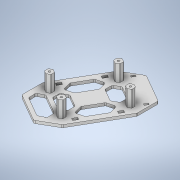
# Autodesk Inventor part: top_body
Saved by Autodesk Inventor 2022 (Build 260153000, 153)
## iProperties
Created: 2022-01-21
Part Number: top_body
Material: Generic
Document SubType Name: Modeling
Designer: felix
Density: 1 g/cm^3
Appearance: Default
Author: felix
Autodesk Inventor part; units mm, degrees
ref_plane "YZ Plane" through (0, 0, 0) normal (1, 0, 0) x (0, 1, 0)
ref_plane "XZ Plane" through (0, 0, 0) normal (0, 1, 0) x (-1, 0, 0)
ref_plane "XY Plane" through (0, 0, 0) normal (0, 0, 1) x (1, 0, 0)
sketch "Sketch1" plane through (0, 0, 0) normal (0, 1, 0) x (-1, 0, 0)
  line L0 (-6.75, 41.2984) -> (6.75, 41.2984)
  line L1 (-8.75, 41.2984) -> (-12.4382, 41.2984)
  line L2 (10.8532, 42.2984) -> (27.4545, 71.0527)
  line L3 (39.1431, 45.1348) -> (-87.6719, 118.3514) construction
  line L4 (27.4545, 73.0527) -> (16.6748, 91.7237)
  line L5 (-8.2836, 49.4226) -> (11.7164, 84.0636) construction
  line L6 (11.7164, 84.0636) -> (-40.2452, 114.0636) construction
  line L7 (-40.2452, 114.0636) -> (-60.2452, 79.4226) construction
  line L8 (-60.2452, 79.4226) -> (-8.2836, 49.4226) construction
  line L9 (27.4545, 73.0527) -> (16.6748, 91.7237)
  line L10 (-13.4382, 41.5663) -> (-38.9549, 56.2984)
  line L11 (15.9428, 92.4557) -> (-9.5739, 107.1878)
  line L12 (-38.9549, 56.2984) -> (-9.5739, 107.1878) construction
  line L13 (8.75, 41.2984) -> (9.1212, 41.2984)
  line L14 (6.75, 41.2984) -> (8.75, 41.2984)
  line L15 (-6.75, 41.2984) -> (-8.75, 41.2984)
  line L16 (-68.0477, 76.6887) -> (-74.7977, 88.38)
  line L17 (-67.0477, 74.9566) -> (-65.2036, 71.7625)
  line L18 (-75.9833, 92.4335) -> (-59.3918, 121.1708)
  line L19 (-57.6613, 122.1708) -> (-36.0921, 122.1878)
  line L20 (-57.6613, 122.1708) -> (-36.0921, 122.1878)
  line L21 (-64.4716, 71.0304) -> (-38.9549, 56.2984)
  line L22 (-35.0906, 121.9198) -> (-9.5739, 107.1878)
  line L23 (-75.7977, 90.1121) -> (-75.9833, 90.4335)
  line L24 (-74.7977, 88.38) -> (-75.7977, 90.1121)
  line L25 (-68.0477, 76.6887) -> (-67.0477, 74.9566)
  line L26 (-41.8469, 122.123) -> (-39.8469, 122.123)
  line L27 (8.363, 47.7877) -> (2.3891, 47.4404)
  line L28 (0.4859, 48.5393) -> (-2.2004, 53.8865)
  line L29 (-2.1453, 55.7843) -> (9.2761, 75.5668)
  line L30 (10.8921, 76.5634) -> (16.8661, 76.9107)
  line L31 (18.7693, 75.8118) -> (21.4556, 70.4646)
  line L32 (21.4005, 68.5668) -> (9.979, 48.7843)
  line L33 (-53.5554, 79.7095) -> (-54.9988, 77.2095)
  line L34 (-55.8648, 76.7095) -> (-58.7516, 76.7095)
  line L35 (-59.6176, 77.2095) -> (-61.061, 79.7095)
  line L36 (-61.061, 80.7095) -> (-59.6176, 83.2095)
  line L37 (-58.7516, 83.7095) -> (-55.8648, 83.7095)
  line L38 (-54.9988, 83.2095) -> (-53.5554, 80.7095)
  circle A0 centre (-57.3082, 80.2095) radius 1.15
  line L39 (-37.1488, 108.1266) -> (-35.7054, 110.6266)
  line L40 (-35.7054, 111.6266) -> (-37.1488, 114.1266)
  line L41 (-38.0148, 114.6266) -> (-40.9016, 114.6266)
  line L42 (-41.7676, 114.1266) -> (-43.211, 111.6266)
  line L43 (-43.211, 110.6266) -> (-41.7676, 108.1266)
  line L44 (-40.9016, 107.6266) -> (-38.0148, 107.6266)
  circle A1 centre (-39.4582, 111.1266) radius 1.15
  line L45 (-11.38, 55.3595) -> (-12.8234, 52.8595)
  line L46 (-12.8234, 51.8595) -> (-11.38, 49.3595)
  line L47 (-10.514, 48.8595) -> (-7.6272, 48.8595)
  line L48 (-6.7612, 49.3595) -> (-5.3178, 51.8595)
  line L49 (-5.3178, 52.8595) -> (-6.7612, 55.3595)
  line L50 (-7.6272, 55.8595) -> (-10.514, 55.8595)
  circle A2 centre (-9.0706, 52.3595) radius 1.15
  line L51 (11.0888, 86.2766) -> (12.5322, 83.7766)
  line L52 (7.336, 86.7766) -> (10.2228, 86.7766)
  line L53 (5.0266, 83.7766) -> (6.47, 86.2766)
  circle A3 centre (8.7794, 83.2766) radius 1.15
  line L54 (12.5322, 82.7766) -> (11.0888, 80.2766)
  line L55 (10.2228, 79.7766) -> (7.336, 79.7766)
  line L56 (6.47, 80.2766) -> (5.0266, 82.7766)
  line L57 (-55.4509, 69.7264) -> (-53.9509, 72.3245)
  line L58 (-53.9509, 72.3245) -> (-49.6208, 69.8245)
  line L59 (-49.6208, 69.8245) -> (-51.1208, 67.2264)
  line L60 (-51.1208, 67.2264) -> (-55.4509, 69.7264)
  line L61 (-29.4509, 114.7598) -> (-30.9509, 112.1617)
  line L62 (-30.9509, 112.1617) -> (-26.6208, 109.6617)
  line L63 (-26.6208, 109.6617) -> (-25.1208, 112.2598)
  line L64 (-25.1208, 112.2598) -> (-29.4509, 114.7598)
  line L65 (-19.0779, 48.7264) -> (-17.5779, 51.3245)
  line L66 (-17.5779, 51.3245) -> (-21.908, 53.8245)
  line L67 (-21.908, 53.8245) -> (-23.408, 51.2264)
  line L68 (-23.408, 51.2264) -> (-19.0779, 48.7264)
  line L69 (2.592, 96.2598) -> (6.9221, 93.7598)
  line L70 (1.092, 93.6617) -> (2.592, 96.2598)
  line L71 (5.4221, 91.1617) -> (1.092, 93.6617)
  line L72 (6.9221, 93.7598) -> (5.4221, 91.1617)
  line L73 (-46.6597, 74.1249) -> (-44.8296, 67.2947)
  line L74 (-43.8977, 66.0803) -> (-28.0121, 56.9088)
  line L75 (-26.4945, 56.709) -> (-19.6643, 58.5391)
  line L76 (-18.2501, 60.9886) -> (-20.0802, 67.8187)
  line L77 (-21.0121, 69.0331) -> (-36.8977, 78.2047)
  line L78 (-38.4154, 78.4045) -> (-45.2455, 76.5744)
  line L79 (18.179, 76.987) -> (1.0762, 47.3641) construction
  line L80 (-47.6152, 61.2984) -> (-30.8618, 90.3161) construction
  line L81 (-30.2946, 51.2984) -> (-13.5413, 80.3161) construction
  line L82 (12.9012, 45.8456) -> (-2.6846, 54.8502) construction
  line L83 (12.8818, 45.8145) -> (-2.6017, 54.7601) construction
  line L84 (-28.8645, 104.9471) -> (-22.0343, 106.7772)
  line L85 (-20.5167, 106.5774) -> (-4.6311, 97.4059)
  line L86 (-3.6992, 96.1914) -> (-1.8691, 89.3613)
  line L87 (-3.2833, 86.9118) -> (-10.1134, 85.0817)
  line L88 (-11.6311, 85.2815) -> (-27.5167, 94.4531)
  line L89 (-28.4486, 95.6675) -> (-30.2787, 102.4976)
  line L90 (-18.2341, 112.1878) -> (-34.9875, 83.1701) construction
  line L91 (-0.9136, 102.1878) -> (-17.667, 73.1701) construction
  line L92 (-57.3082, 80.2095) -> (8.7794, 83.2766) construction
  line L93 (-9.0706, 52.3595) -> (-39.4582, 111.1266) construction
  line L94 (-17.7325, 59.0567) -> (-47.1773, 76.0567) construction
  line L95 (-1.3515, 87.4295) -> (-30.7963, 104.4295) construction
  line L96 (-52.6301, 88.8824) -> (-40.5057, 81.8824) construction
  line L97 (-44.6301, 102.7388) -> (-32.5057, 95.7388) construction
  line L98 (-36.5978, 102.6513) -> (-48.5381, 81.97) construction
  line L99 (3.5167, 73.5911) -> (-3.3141, 61.76)
  line L100 (-5.0679, 60.7601) -> (-10.8053, 60.8227)
  line L101 (-12.5045, 61.8037) -> (-15.4274, 66.7411)
  line L102 (-15.4384, 68.76) -> (-8.6077, 80.5911)
  line L103 (-6.8538, 81.591) -> (-1.1165, 81.5284)
  line L104 (0.5828, 80.5474) -> (3.5057, 75.6099)
  line L105 (-3.8987, 60.7473) -> (-16.0231, 67.7473) construction
  line L106 (4.1013, 74.6038) -> (-8.0231, 81.6038) construction
  line L107 (0.0093, 81.5162) -> (-11.931, 60.8349) construction
  arc A4 (-57.6613, 122.1708) -> (-59.3918, 121.1708) centre (-57.6598, 120.1708) ccw
  arc A5 (-75.9833, 92.4335) -> (-75.9833, 90.4335) centre (-74.2513, 91.4335) ccw
  arc A6 (-35.0906, 121.9198) -> (-36.0921, 122.1878) centre (-36.0906, 120.1878) ccw
  arc A7 (16.6748, 91.7237) -> (15.9428, 92.4557) centre (14.9428, 90.7237) ccw
  arc A8 (27.4545, 71.0527) -> (27.4545, 73.0527) centre (25.7225, 72.0527) ccw
  arc A9 (9.1212, 41.2984) -> (10.8532, 42.2984) centre (9.1212, 43.2984) ccw
  arc A10 (-13.4382, 41.5663) -> (-12.4382, 41.2984) centre (-12.4382, 43.2984) ccw
  arc A11 (-65.2036, 71.7625) -> (-64.4716, 71.0304) centre (-63.4716, 72.7625) ccw
  arc A12 (-61.061, 80.7095) -> (-61.061, 79.7095) centre (-60.195, 80.2095) ccw
  arc A13 (-58.7516, 83.7095) -> (-59.6176, 83.2095) centre (-58.7516, 82.7095) ccw
  arc A14 (-54.9988, 83.2095) -> (-55.8648, 83.7095) centre (-55.8648, 82.7095) ccw
  arc A15 (-53.5554, 79.7095) -> (-53.5554, 80.7095) centre (-54.4215, 80.2095) ccw
  arc A16 (-55.8648, 76.7095) -> (-54.9988, 77.2095) centre (-55.8648, 77.7095) ccw
  arc A17 (-59.6176, 77.2095) -> (-58.7516, 76.7095) centre (-58.7516, 77.7095) ccw
  arc A18 (-43.211, 111.6266) -> (-43.211, 110.6266) centre (-42.345, 111.1266) ccw
  arc A19 (-40.9016, 114.6266) -> (-41.7676, 114.1266) centre (-40.9016, 113.6266) ccw
  arc A20 (-37.1488, 114.1266) -> (-38.0148, 114.6266) centre (-38.0148, 113.6266) ccw
  arc A21 (-35.7054, 110.6266) -> (-35.7054, 111.6266) centre (-36.5715, 111.1266) ccw
  arc A22 (-38.0148, 107.6266) -> (-37.1488, 108.1266) centre (-38.0148, 108.6266) ccw
  arc A23 (-41.7676, 108.1266) -> (-40.9016, 107.6266) centre (-40.9016, 108.6266) ccw
  arc A24 (7.336, 86.7766) -> (6.47, 86.2766) centre (7.336, 85.7766) ccw
  arc A25 (11.0888, 86.2766) -> (10.2228, 86.7766) centre (10.2228, 85.7766) ccw
  arc A26 (12.5322, 82.7766) -> (12.5322, 83.7766) centre (11.6662, 83.2766) ccw
  arc A27 (10.2228, 79.7766) -> (11.0888, 80.2766) centre (10.2228, 80.7766) ccw
  arc A28 (6.47, 80.2766) -> (7.336, 79.7766) centre (7.336, 80.7766) ccw
  arc A29 (5.0266, 83.7766) -> (5.0266, 82.7766) centre (5.8927, 83.2766) ccw
  arc A30 (-12.8234, 52.8595) -> (-12.8234, 51.8595) centre (-11.9573, 52.3595) ccw
  arc A31 (-11.38, 49.3595) -> (-10.514, 48.8595) centre (-10.514, 49.8595) ccw
  arc A32 (-7.6272, 48.8595) -> (-6.7612, 49.3595) centre (-7.6272, 49.8595) ccw
  arc A33 (-5.3178, 51.8595) -> (-5.3178, 52.8595) centre (-6.1838, 52.3595) ccw
  arc A34 (-6.7612, 55.3595) -> (-7.6272, 55.8595) centre (-7.6272, 54.8595) ccw
  arc A35 (-10.514, 55.8595) -> (-11.38, 55.3595) centre (-10.514, 54.8595) ccw
  arc A36 (-45.2455, 76.5744) -> (-46.6597, 74.1249) centre (-44.7278, 74.6425) ccw
  arc A37 (-36.8977, 78.2047) -> (-38.4154, 78.4045) centre (-37.8977, 76.4726) ccw
  arc A38 (-44.8296, 67.2947) -> (-43.8977, 66.0803) centre (-42.8977, 67.8124) ccw
  arc A39 (-28.0121, 56.9088) -> (-26.4945, 56.709) centre (-27.0121, 58.6408) ccw
  arc A40 (-19.6643, 58.5391) -> (-18.2501, 60.9886) centre (-20.182, 60.4709) ccw
  arc A41 (-20.0802, 67.8187) -> (-21.0121, 69.0331) centre (-22.0121, 67.3011) ccw
  arc A42 (-28.4486, 95.6675) -> (-27.5167, 94.4531) centre (-26.5167, 96.1851) ccw
  arc A43 (-28.8645, 104.9471) -> (-30.2787, 102.4976) centre (-28.3468, 103.0153) ccw
  arc A44 (-20.5167, 106.5774) -> (-22.0343, 106.7772) centre (-21.5167, 104.8454) ccw
  arc A45 (-3.6992, 96.1914) -> (-4.6311, 97.4059) centre (-5.6311, 95.6738) ccw
  arc A46 (-3.2833, 86.9118) -> (-1.8691, 89.3613) centre (-3.801, 88.8437) ccw
  arc A47 (-11.6311, 85.2815) -> (-10.1134, 85.0817) centre (-10.6311, 87.0136) ccw
  arc A48 (-2.1453, 55.7843) -> (-2.2004, 53.8865) centre (-0.4133, 54.7843) ccw
  arc A49 (10.8921, 76.5634) -> (9.2761, 75.5668) centre (11.0082, 74.5668) ccw
  arc A50 (18.7693, 75.8118) -> (16.8661, 76.9107) centre (16.9821, 74.914) ccw
  arc A51 (21.4005, 68.5668) -> (21.4556, 70.4646) centre (19.6684, 69.5668) ccw
  arc A52 (8.363, 47.7877) -> (9.979, 48.7843) centre (8.247, 49.7843) ccw
  arc A53 (0.4859, 48.5393) -> (2.3891, 47.4404) centre (2.273, 49.4371) ccw
  arc A54 (-15.4384, 68.76) -> (-15.4274, 66.7411) centre (-13.7064, 67.76) ccw
  arc A55 (-6.8538, 81.591) -> (-8.6077, 80.5911) centre (-6.8756, 79.5911) ccw
  arc A56 (0.5828, 80.5474) -> (-1.1165, 81.5284) centre (-1.1383, 79.5286) ccw
  arc A57 (3.5167, 73.5911) -> (3.5057, 75.6099) centre (1.7846, 74.5911) ccw
  arc A58 (-5.0679, 60.7601) -> (-3.3141, 61.76) centre (-5.0461, 62.76) ccw
  arc A59 (-12.5045, 61.8037) -> (-10.8053, 60.8227) centre (-10.7835, 62.8225) ccw
  line L108 (-45.2147, 101.7262) -> (-52.0455, 89.8951)
  line L109 (-52.0345, 87.8762) -> (-49.1116, 82.9388)
  line L110 (-47.4123, 81.9577) -> (-41.675, 81.8952)
  line L111 (-37.7235, 102.6635) -> (-43.4609, 102.7261)
  line L112 (-33.1014, 96.745) -> (-36.0243, 101.6825)
  line L113 (-39.9211, 82.8951) -> (-33.0904, 94.7262)
  arc A60 (-41.675, 81.8952) -> (-39.9211, 82.8951) centre (-41.6532, 83.8951) ccw
  arc A61 (-33.0904, 94.7262) -> (-33.1014, 96.745) centre (-34.8224, 95.7262) ccw
  arc A62 (-36.0243, 101.6825) -> (-37.7235, 102.6635) centre (-37.7453, 100.6636) ccw
  arc A63 (-43.4609, 102.7261) -> (-45.2147, 101.7262) centre (-43.4827, 100.7262) ccw
  arc A64 (-52.0455, 89.8951) -> (-52.0345, 87.8762) centre (-50.3134, 88.8951) ccw
  arc A65 (-49.1116, 82.9388) -> (-47.4123, 81.9577) centre (-47.3905, 83.9576) ccw
  point P0 (10.2759, 41.2984)
  point P1 (-12.9741, 41.2984)
  point P2 (28.0319, 72.0527)
  point P3 (19.1539, 56.6755)
  point P4 (-67.6827, 106.8106)
  point P5 (-8.2836, 49.4226)
  point P6 (-24.2644, 81.7431)
  point P7 (9.4398, 47.8502)
  point P8 (21.9398, 69.5009)
  point P9 (-53.2668, 80.2095)
  point P10 (-55.2875, 76.7095)
  point P11 (-59.3289, 76.7095)
  point P12 (-61.3497, 80.2095)
  point P13 (-59.3289, 83.7095)
  point P14 (-55.2875, 83.7095)
  point P15 (-37.4375, 107.6266)
  point P16 (-35.4168, 111.1266)
  point P17 (-37.4375, 114.6266)
  point P18 (-41.4789, 114.6266)
  point P19 (-43.4997, 111.1266)
  point P20 (-41.4789, 107.6266)
  point P21 (-11.0913, 55.8595)
  point P22 (-13.112, 52.3595)
  point P23 (-11.0913, 48.8595)
  point P24 (-7.0499, 48.8595)
  point P25 (-5.0291, 52.3595)
  point P26 (-7.0499, 55.8595)
  point P27 (10.8001, 86.7766)
  point P28 (12.8209, 83.2766)
  point P29 (6.7587, 86.7766)
  point P30 (4.738, 83.2766)
  point P31 (10.8001, 79.7766)
  point P32 (6.7587, 79.7766)
  point P33 (-44.6152, 66.4945)
  point P34 (-27.2946, 56.4945)
  point P35 (-20.2946, 68.6189)
  point P36 (-37.6152, 78.6189)
  point P37 (-21.2341, 106.9916)
  point P38 (-3.9136, 96.9916)
  point P39 (-10.9136, 84.8673)
  point P40 (-28.2341, 94.8673)
  dimension "d82" = 23.25
  dimension "d88" = 120
  dimension "d89" = 120
  dimension "d90" = 35.512
  dimension "d91" = 17.756
  dimension "d92" = 17.756
  dimension "d95" = 40
  dimension "d97" = 20
  dimension "d99" = 30
  dimension "d102" = 60
  dimension "d145" = 180
  dimension "d146" = 30
  dimension "d147" = 8.1242
  dimension "d148" = 8.1242
  dimension "d155" = 2.3
  dimension "d156" = 7
  dimension "d160" = 3
  dimension "d162" = 3
  dimension "d163" = 9
  dimension "d169" = 6
  dimension "d170" = 10
  dimension "d171" = 20
  dimension "d172" = 14
  dimension "d179" = 7
  dimension "d181" = 2
  dimension "d186" = 1
  dimension "d187" = 1
  dimension "d189" = 2
  dimension "d190" = 2
  dimension "d191" = 4
  dimension "d192" = 16
  dimension "d193" = 8
  dimension "d194" = 14
  dimension "d195" = 8
  dimension "d204" = 14
  dimension "d206" = 18.762
  dimension "d207" = 28.2702
  dimension "d238" = 5
  dimension "d244" = 25
  dimension "d245" = 12.5
  dimension "d246" = 0
  dimension "d247" = 4
  dimension "d275" = 2.15
  dimension "d276" = 2.15
  constraints: 228 end point, 124 point on circle, 112 tangent, 110 point on line, 79 symmetric about line, 66 centre point, 51 equal radius, 16 parallel, 9 equal length, 6 perpendicular, 4 collinear, 3 coincident, 3 midpoint, 2 horizontal, 22 other
  measures "d82" distance of point (10.276, 41.298) point (-12.974, 41.298)
  measures "d88" angle of L2 L1
  measures "d89" angle of L4 L2
  measures "d90" distance of point (10.276, 41.298) point (28.032, 72.053)
  measures "d91" distance of point (19.154, 56.676) point (10.276, 41.298)
  measures "d92" distance of point (28.032, 72.053) point (19.154, 56.676)
  measures "d95" distance of L5.start L5.end
  measures "d97" distance from line of L3 L5.start
  measures "d99" distance of L10.end point (-12.974, 41.298)
  measures "d102" distance of L7.end L5.start
  measures "d145" angle of L10 L21
  measures "d146" distance from line of L5 point (-24.264, 81.743)
  measures "d147" distance from line of L0 L5.start
  measures "d148" distance from line of L4 L5.end
  measures "d155" diameter of A0
  measures "d156" distance between parallel lines of L38 L35
  measures "d160" distance between parallel lines of L58 L60
  measures "d162" distance between parallel lines of L8 L58
  measures "d163" distance between parallel lines of L57 L7
  measures "d169" distance between parallel lines of L21 L74
  measures "d170" distance from line of L12 point (-27.295, 56.495)
  measures "d171" distance of point (-44.615, 66.495) point (-27.295, 56.495)
  measures "d172" distance between parallel lines of L77 L74
  measures "d179" distance from line of L94.end L80
  measures "d181" radius of A4
  measures "d186" radius of A12
  measures "d187" radius of A27
  measures "d189" radius of A36
  measures "d190" radius of A54
  measures "d191" distance between parallel lines of L29 L99
  measures "d192" distance of L105.start L106.start
  measures "d193" distance from line of L3 L106.start
  measures "d194" distance between parallel lines of L99 L102
  measures "d195" distance between parallel lines of L106 L3
  measures "d204" distance between parallel lines of L32 L29
  measures "d206" distance between parallel lines of L88 L77
  measures "d207" distance between parallel lines of L113 L102
  measures "d238" distance of L59.end L57.start
  measures "d244" distance of point (21.94, 69.501) point (9.44, 47.85)
  measures "d245" distance from line of L3 point (9.44, 47.85)
  measures "d246" angle of L83 L82
  measures "d247" distance between parallel lines of L2 L32
  measures "d275" distance from line of L92.start L7
  measures "d276" distance from line of L8 point (-57.308, 80.21)
extrude "Extrusion1_main_body" add sketch "Sketch1" along normal blind 3 contours L15 L1 A10 L10 L21 A11 L17 L25 L16 L24 L23 A5 L18 A4 L19 A6 L22 L11 A7 L4 A8 L2 A9 L13 L14 L0
extrude "Extrusion2_main_body" add sketch "Sketch1" along normal blind 21 contours L33 A16 L34 A17 L35 A12 L36 A13 L37 A14 L38 A15 | A22 L44 A23 L43 A18 L42 A19 L41 A20 L40 A21 L39 | A35 L50 A34 L49 A33 L48 A32 L47 A31 L46 A30 L45 | L51 A26 L54 A27 L55 A28 L56 A29 L53 A24 L52 A25
extrude "Extrusion3_main_body" add sketch "Sketch1" along normal blind 13 contours A0 | A1 | A2 | A3
sketch "Sketch2_insert" plane through (0, 0, 0) normal (0, -1, 0) x (1, 0, 0)
  line L0 (43.6302, 119.4707) -> (66.6302, 79.6336)
  line L1 (66.6302, 79.6336) -> (65.0713, 78.7336)
  line L2 (65.0713, 78.7336) -> (42.0713, 118.5707)
  line L3 (42.0713, 118.5707) -> (43.6302, 119.4707)
  line L4 (59.3918, 121.1708) -> (75.9833, 92.4335) projected
  line L5 (52.0455, 89.8951) -> (45.2147, 101.7262) projected
  line L6 (64.4716, 71.0304) -> (13.4382, 41.5663) projected
  line L7 (-15.9428, 92.4557) -> (35.0906, 121.9198) projected
  line L8 (66.7221, 106.2448) -> (52.3926, 97.9716) construction
  line L9 (59.3918, 121.1708) -> (75.9833, 92.4335) projected
  line L10 (51.0713, 102.9823) -> (47.3474, 100.8323)
  line L11 (47.3474, 100.8323) -> (52.3474, 92.172)
  line L12 (52.3474, 92.172) -> (56.0713, 94.322)
  line L13 (52.6358, 103.8726) -> (54.6276, 105.0226)
  line L14 (54.6276, 105.0226) -> (59.6276, 96.3624)
  line L15 (59.6276, 96.3624) -> (57.6358, 95.2124)
  line L16 (46.9453, 118.7289) -> (50.4094, 120.7289)
  line L17 (50.4094, 120.7289) -> (51.4094, 118.9968)
  line L18 (51.4094, 118.9968) -> (47.9453, 116.9968)
  line L19 (47.9453, 116.9968) -> (46.9453, 118.7289)
  line L20 (36.0921, 122.1878) -> (57.6613, 122.1708) projected
  line L21 (67.6453, 82.8754) -> (71.1094, 84.8754)
  line L22 (71.1094, 84.8754) -> (70.1094, 86.6075)
  line L23 (70.1094, 86.6075) -> (66.6453, 84.6075)
  line L24 (66.6453, 84.6075) -> (67.6453, 82.8754)
  point P0 (0, 0)
  point P1 (55.1302, 99.5522)
  point P2 (67.6876, 106.8022)
  point P3 (49.8474, 96.5022)
  dimension "d249" = 1.8
  dimension "d251" = 46
  dimension "d252" = 23
  dimension "d254" = 10
  dimension "d255" = 4.3
  dimension "d256" = 1.4
  dimension "d258" = 2.3
  dimension "d265" = 4
  dimension "d266" = 2
  dimension "d267" = 2.5
  dimension "d268" = 2.3
  dimension "d269" = 1.4477
  dimension "d272" = 8
  dimension "d273" = 10
  constraints: 38 end point, 12 parallel, 7 point on line, 6 perpendicular, 4 symmetric about line, 3 midpoint
  measures "d249" distance of L2.end L0.start
  measures "d251" distance of L0.start L0.end
  measures "d252" distance of L0.start point (55.13, 99.552)
  measures "d254" distance between parallel lines of L12 L10
  measures "d255" distance of L11.end L12.end
  measures "d256" distance between parallel lines of L5 L11
  measures "d258" distance of L13.start L13.end
  measures "d265" distance of L16.start L16.end
  measures "d266" distance between parallel lines of L18 L16
  measures "d267" distance between parallel lines of L0 L19
  measures "d268" distance between parallel lines of L16 L3
  measures "d269" distance from line of L16.end L20
  measures "d272" distance between parallel lines of L17 L4
  measures "d273" distance between parallel lines of L15 L13
extrude "Extrusion1_feature1" cut sketch "Sketch2_insert" against normal blind 1.5 contours L0 L1 L2 L3
extrude "Extrusion2_feature1" cut sketch "Sketch2_insert" against normal blind 1.2 contours L13 L14 L15 L0
extrude "Extrusion3_feature1" cut sketch "Sketch2_insert" against normal blind 3 contours L2 L12 L11 L10
extrude "Extrusion4_feature1_zip_ties" cut sketch "Sketch2_insert" against normal blind 3 contours L16 L17 L18 L19 | L24 L23 L22 L21
body "Solid1"
